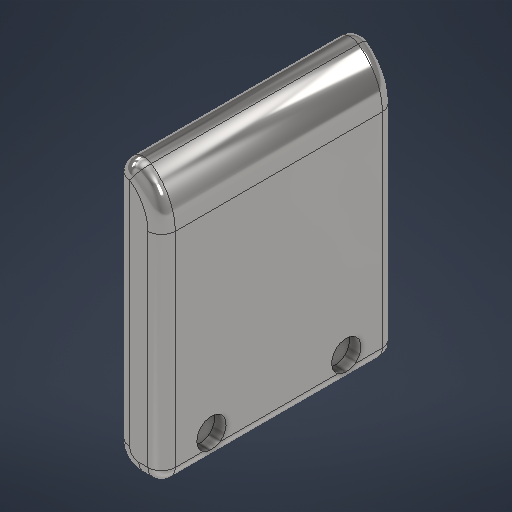
# Autodesk Inventor part: back
Saved by Autodesk Inventor 2027 (Build 310192000, 192)
## iProperties
Created: 2026-04-25
Part Number: back
Material: Sherpa
Document SubType Name: Modeling
Designer: sisis
Density: 0.9 g/cm^3
Appearance: Stripes - Black-White-Blue-Gray 1(1)
Author: sisis
Autodesk Inventor part; units mm, degrees
ref_plane "YZ Plane" through (0, 0, 0) normal (1, 0, 0) x (0, 1, 0)
ref_plane "XZ Plane" through (0, 0, 0) normal (0, 1, 0) x (-1, 0, 0)
ref_plane "XY Plane" through (0, 0, 0) normal (0, 0, 1) x (1, 0, 0)
sketch "Sketch1" plane through (0, 0, 0) normal (1, 0, 0) x (0, 1, 0)
  line L0 (0, 0) -> (12.7529, 0)
  line L1 (0, 0) -> (12.7529, 0)
  line L2 (0, 0) -> (15.2283, 0)
  line L3 (15.2283, 0) -> (15.2283, -13.0243)
  line L4 (15.2283, -13.0243) -> (0, -13.0243)
  line L5 (0, -13.0243) -> (0, 0)
  dimension "d13" = 13.0243
  constraints: 12 end point, 3 perpendicular, 2 horizontal, 1 collinear
  measures "d13" distance of L4.end L0.start
extrude "Extrusion1" add sketch "Sketch1" along normal blind 2.54
fillet "Fillet1" radius 3.175 1 edges at (2.54, 15.2283, -6.5121)
sketch "Sketch2" plane through (2.54, 0, 0) normal (1, 0, 0) x (0, 0, -1)
  circle A0 centre (2.7686, 1.4224) radius 0.8128
  line L0 (0, 12.1174) -> (0, 0) projected
  line L1 (0, 0) -> (13.0243, 0) projected
  circle A1 centre (10.2557, 1.4224) radius 0.8128
  line L2 (13.0243, 0) -> (13.0243, 15.2283) projected
  dimension "d4" = 1.6256
  dimension "d5" = 2.7686
  dimension "d6" = 1.4224
  dimension "d7" = 1.6256
  dimension "d8" = 2.7686
  dimension "d9" = 1.4224
  constraints: 2 centre point
  measures "d4" diameter of A0
  measures "d5" distance from line of A0.centre L0
  measures "d6" distance from line of A0.centre L1
  measures "d7" diameter of A1
  measures "d8" distance from line of A1.centre L2
  measures "d9" distance from line of L1 A1.centre
extrude "Extrusion2" cut sketch "Sketch2" against normal blind 0.635
fillet "Fillet2" radius 1.27 1 edges at (0, 0, -6.5121)
fillet "Fillet3" radius 0.762 1 edges at (0, 15.2283, -6.5121)
fillet "Fillet4" radius 0.762 6 edges at (2.54, 6.0587, -13.0243) (2.1861, 13.5742, -13.0243) (0.4124, 14.762, -13.0243) (0, 7.6774, -13.0243) (0.372, 0.372, -13.0243) (1.905, 0, -13.0243)
fillet "Fillet5" radius 0.762 8 edges at (2.54, 0, -6.1311) (2.3168, 0.2232, -12.8011) (2.1861, 13.5742, 0) (0.4124, 14.762, 0) (0, 7.6774, 0) (0.372, 0.372, 0) (1.905, 0, 0) (2.54, 6.0587, 0)
body "Solid1"
